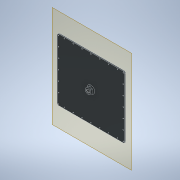
# Autodesk Inventor part: Крышка картера 2
Saved by Autodesk Inventor 2021 (Build 250183000, 183)
## iProperties
Created: 2020-12-12
Part Number: Крышка картера 2
Material: Чугун, серый
Document SubType Name: Modeling
Designer: Тимоха
Mass: 32984 g
Surface Area: 9566.62 cm^2
Volume: 4613.15 cm^3
Density: 7.15 g/cm^3
Appearance: Чугун серый
Author: Тимоха
Autodesk Inventor part; units mm, degrees
ref_plane "YZ Plane" through (0, 0, 0) normal (1, 0, 0) x (0, 1, 0)
ref_plane "XZ Plane" through (0, 0, 0) normal (0, 1, 0) x (-1, 0, 0)
ref_plane "XY Plane" through (0, 0, 0) normal (0, 0, 1) x (1, 0, 0)
ref_plane "РабПлоскость1" through (0, 0, 0) normal (0, 0, 1) x (1, 0, 0)
sketch "Эскиз1" plane through (0, 0, 0) normal (0, 0, 1) x (1, 0, 0)
  circle A0 centre (340, 472) radius 4 projected
  circle A1 centre (340, 367) radius 4 projected
  circle A2 centre (340, 322.8) radius 4 projected
  circle A3 centre (340, 218.5) radius 4 projected
  circle A4 centre (340, 114.2) radius 4 projected
  circle A5 centre (340, 9.9) radius 4 projected
  circle A6 centre (340, -94.4) radius 4 projected
  circle A7 centre (340, -198.7) radius 4 projected
  circle A8 centre (340, -303) radius 4 projected
  circle A9 centre (340, -347) radius 4 projected
  circle A10 centre (340, -407) radius 4 projected
  circle A11 centre (340, -467) radius 4 projected
  circle A12 centre (278, 472) radius 4 projected
  circle A13 centre (185, 472) radius 4 projected
  circle A14 centre (92, 472) radius 4 projected
  circle A15 centre (-1, 472) radius 4 projected
  circle A16 centre (-94, 472) radius 4 projected
  circle A17 centre (-187, 472) radius 4 projected
  circle A18 centre (-280, 472) radius 4 projected
  circle A19 centre (-340, 472) radius 4 projected
  circle A20 centre (-340, 367) radius 4 projected
  circle A21 centre (-340, 322.8) radius 4 projected
  circle A22 centre (-340, 218.5) radius 4 projected
  circle A23 centre (-340, 114.2) radius 4 projected
  circle A24 centre (-340, 9.9) radius 4 projected
  circle A25 centre (-340, -94.4) radius 4 projected
  circle A26 centre (-340, -198.7) radius 4 projected
  circle A27 centre (-340, -303) radius 4 projected
  circle A28 centre (-340, -347) radius 4 projected
  circle A29 centre (-340, -407) radius 4 projected
  circle A30 centre (-340, -467) radius 4 projected
  line L0 (165, -460) -> (165, -485) projected
  line L1 (185, -485) -> (165, -485) projected
  line L2 (185, -475) -> (185, -485) projected
  line L3 (185, -475) -> (380, -475) projected
  line L4 (380, 475) -> (350, 475) projected
  line L5 (350, 475) -> (350, 485) projected
  line L6 (-350, 485) -> (350, 485) projected
  line L7 (-350, 475) -> (-350, 485) projected
  line L8 (-350, 475) -> (-380, 475) projected
  line L9 (-380, -475) -> (-185, -475) projected
  line L10 (-185, -475) -> (-185, -485) projected
  line L11 (-165, -485) -> (-185, -485) projected
  line L12 (-165, -485) -> (-165, -460) projected
  line L13 (-165, -460) -> (-330, -460) projected
  line L14 (-330, 460) -> (-330, -460) projected
  line L15 (-330, 460) -> (330, 460) projected
  line L16 (330, -460) -> (330, 460) projected
  line L17 (330, -460) -> (165, -460) projected
  circle A31 centre (278, -303) radius 4 projected
  circle A32 centre (185, -303) radius 4 projected
  circle A33 centre (92, -303) radius 4 projected
  circle A34 centre (-1, -303) radius 4 projected
  circle A35 centre (-94, -303) radius 4 projected
  circle A36 centre (-187, -303) radius 4 projected
  circle A37 centre (-280, -303) radius 4 projected
  circle A38 centre (278, -347) radius 4 projected
  circle A39 centre (185, -347) radius 4 projected
  circle A40 centre (92, -347) radius 4 projected
  circle A41 centre (-1, -347) radius 4 projected
  circle A42 centre (-94, -347) radius 4 projected
  circle A43 centre (-187, -347) radius 4 projected
  circle A44 centre (-280, -347) radius 4 projected
  line L18 (-330, -291) -> (-330, -359) projected
  line L19 (-330, -359) -> (330, -359) projected
  line L20 (330, -291) -> (330, -359) projected
  line L21 (-330, -291) -> (330, -291) projected
  circle A45 centre (278, 367) radius 4 projected
  circle A46 centre (185, 367) radius 4 projected
  circle A47 centre (92, 367) radius 4 projected
  circle A48 centre (-1, 367) radius 4 projected
  circle A49 centre (-94, 367) radius 4 projected
  circle A50 centre (-187, 367) radius 4 projected
  circle A51 centre (-280, 367) radius 4 projected
  circle A52 centre (278, 323) radius 4 projected
  circle A53 centre (185, 323) radius 4 projected
  circle A54 centre (92, 323) radius 4 projected
  circle A55 centre (-1, 323) radius 4 projected
  circle A56 centre (-94, 323) radius 4 projected
  circle A57 centre (-187, 323) radius 4 projected
  circle A58 centre (-280, 323) radius 4 projected
  line L22 (-330, 379) -> (-330, 311) projected
  line L23 (-330, 311) -> (330, 311) projected
  line L24 (330, 379) -> (330, 311) projected
  line L25 (-330, 379) -> (330, 379) projected
  circle A59 centre (-340, 322.8) radius 14
  circle A60 centre (-340, -303) radius 14
  circle A61 centre (340, -303) radius 14
  circle A62 centre (340, 322.8) radius 14
  line L26 (340, 336.8) -> (-340, 336.8)
  line L27 (-354, 322.8) -> (-354, -303)
  line L28 (-340, -317) -> (340, -317)
  line L29 (354, -303) -> (354, 322.8)
  spline S0 degree 3 poles (-370, 316.7157) (-371.226, 316.7157) (-372.452, 316.5956) (-375.5798, 315.9798) (-377.4441, 315.3011) (-379.4493, 314.2131) (-379.7267, 314.0539) (-380, 313.8881) knots 25.431649 25.431649 25.431649 25.431649 25.799448 25.799448 26.387926 26.387926 26.483827 26.483827 26.483827 26.483827 projected
  spline S1 degree 3 poles (-360, 299.3952) (-360, 300.6696) (-360.1945, 302.0462) (-360.9458, 304.7063) (-361.4997, 305.9906) (-363.0323, 308.8381) (-364.2894, 310.5672) (-367.0866, 313.808) (-368.6145, 315.3302) (-370, 316.7157) knots 0 0 0 0 0.382316 0.382316 0.764632 0.764632 1.352446 1.352446 1.94026 1.94026 1.94026 1.94026 projected
  line L30 (-360, 299.3952) -> (-360, 277.9108) projected
  spline S2 degree 3 poles (-370, 260.5903) (-368.6145, 261.9758) (-367.0866, 263.498) (-364.2894, 266.7388) (-363.0323, 268.4679) (-361.4997, 271.3154) (-360.9458, 272.5997) (-360.1945, 275.2598) (-360, 276.6364) (-360, 277.9108) knots 5.055322 5.055322 5.055322 5.055322 5.643136 5.643136 6.230951 6.230951 6.613267 6.613267 6.995583 6.995583 6.995583 6.995583 projected
  spline S3 degree 3 poles (-380, 263.2891) (-378.6731, 262.5173) (-377.2567, 261.8994) (-373.9153, 260.8819) (-371.9577, 260.5903) (-370, 260.5903) knots 11.600008 11.600008 11.600008 11.600008 12.060517 12.060517 12.64782 12.64782 12.64782 12.64782 projected
  line L31 (-380, 263.2891) -> (-380, -243.2891) projected
  spline S4 degree 3 poles (-370, -240.5903) (-371.2894, -240.5903) (-372.5789, -240.7163) (-375.8683, -241.3651) (-377.8293, -242.082) (-379.7569, -243.1494) (-379.8788, -243.2186) (-380, -243.2891) knots 12.64782 12.64782 12.64782 12.64782 13.034648 13.034648 13.653574 13.653574 13.695631 13.695631 13.695631 13.695631 projected
  spline S5 degree 3 poles (-360, -257.9108) (-360, -256.6364) (-360.1945, -255.2598) (-360.9458, -252.5997) (-361.4997, -251.3154) (-363.0323, -248.4679) (-364.2894, -246.7388) (-367.0866, -243.498) (-368.6145, -241.9758) (-370, -240.5903) knots 0 0 0 0 0.382316 0.382316 0.764632 0.764632 1.352446 1.352446 1.94026 1.94026 1.94026 1.94026 projected
  line L32 (-360, -257.9108) -> (-360, -279.3952) projected
  spline S6 degree 3 poles (-370, -296.7157) (-368.6145, -295.3302) (-367.0866, -293.808) (-364.2894, -290.5672) (-363.0323, -288.8381) (-361.4997, -285.9906) (-360.9458, -284.7063) (-360.1945, -282.0462) (-360, -280.6696) (-360, -279.3952) knots 5.055322 5.055322 5.055322 5.055322 5.643136 5.643136 6.230951 6.230951 6.613267 6.613267 6.995583 6.995583 6.995583 6.995583 projected
  spline S7 degree 3 poles (-380, -293.8881) (-379.7267, -294.0539) (-379.4493, -294.2131) (-377.4441, -295.3011) (-375.5798, -295.9798) (-372.452, -296.5956) (-371.226, -296.7157) (-370, -296.7157) knots -1.052177 -1.052177 -1.052177 -1.052177 -0.956277 -0.956277 -0.367799 -0.367799 0 0 0 0 projected
  line L33 (-380, -293.8881) -> (-380, -356.1119) projected
  spline S8 degree 3 poles (-370, -353.2843) (-371.226, -353.2843) (-372.452, -353.4044) (-375.5798, -354.0202) (-377.4441, -354.6989) (-379.4493, -355.7869) (-379.7267, -355.9461) (-380, -356.1119) knots 12.715825 12.715825 12.715825 12.715825 13.083623 13.083623 13.672101 13.672101 13.768002 13.768002 13.768002 13.768002 projected
  spline S9 degree 3 poles (-360, -370.6048) (-360, -369.3304) (-360.1945, -367.9538) (-360.9458, -365.2937) (-361.4997, -364.0094) (-363.0323, -361.1619) (-364.2894, -359.4328) (-367.0866, -356.192) (-368.6145, -354.6698) (-370, -353.2843) knots 0 0 0 0 0.382316 0.382316 0.764632 0.764632 1.352446 1.352446 1.94026 1.94026 1.94026 1.94026 projected
  line L34 (-360, -370.6048) -> (-360, -392.0892) projected
  spline S10 degree 3 poles (-370, -409.4097) (-368.6145, -408.0242) (-367.0866, -406.502) (-364.2894, -403.2612) (-363.0323, -401.5321) (-361.4997, -398.6846) (-360.9458, -397.4003) (-360.1945, -394.7402) (-360, -393.3636) (-360, -392.0892) knots 5.055322 5.055322 5.055322 5.055322 5.643136 5.643136 6.230951 6.230951 6.613267 6.613267 6.995583 6.995583 6.995583 6.995583 projected
  spline S11 degree 3 poles (-380, -406.7109) (-379.8788, -406.7814) (-379.7569, -406.8506) (-377.8293, -407.918) (-375.8683, -408.6349) (-372.5789, -409.2837) (-371.2894, -409.4097) (-370, -409.4097) knots -1.047812 -1.047812 -1.047812 -1.047812 -1.005754 -1.005754 -0.386829 -0.386829 0 0 0 0 projected
  line L35 (-380, -406.7109) -> (-380, -475) projected
  line L36 (380, -475) -> (380, -406.7109) projected
  spline S12 degree 3 poles (370, -409.4097) (371.2894, -409.4097) (372.5789, -409.2837) (375.8683, -408.6349) (377.8293, -407.918) (379.7569, -406.8506) (379.8788, -406.7814) (380, -406.7109) knots 12.64782 12.64782 12.64782 12.64782 13.034648 13.034648 13.653574 13.653574 13.695631 13.695631 13.695631 13.695631 projected
  spline S13 degree 3 poles (360, -392.0892) (360, -393.3636) (360.1945, -394.7402) (360.9458, -397.4003) (361.4997, -398.6846) (363.0323, -401.5321) (364.2894, -403.2612) (367.0866, -406.502) (368.6145, -408.0242) (370, -409.4097) knots 0 0 0 0 0.382316 0.382316 0.764632 0.764632 1.352446 1.352446 1.94026 1.94026 1.94026 1.94026 projected
  line L37 (360, -392.0892) -> (360, -370.6048) projected
  spline S14 degree 3 poles (370, -353.2843) (368.6145, -354.6698) (367.0866, -356.192) (364.2894, -359.4328) (363.0323, -361.1619) (361.4997, -364.0094) (360.9458, -365.2937) (360.1945, -367.9538) (360, -369.3304) (360, -370.6048) knots 5.055322 5.055322 5.055322 5.055322 5.643136 5.643136 6.230951 6.230951 6.613267 6.613267 6.995583 6.995583 6.995583 6.995583 projected
  spline S15 degree 3 poles (380, -356.1119) (378.2451, -355.0477) (376.3252, -354.255) (372.9103, -353.4538) (371.4552, -353.2843) (370, -353.2843) knots -1.052177 -1.052177 -1.052177 -1.052177 -0.436564 -0.436564 0 0 0 0 projected
  line L38 (380, -356.1119) -> (380, -293.8881) projected
  spline S16 degree 3 poles (370, -296.7157) (371.226, -296.7157) (372.452, -296.5956) (375.5798, -295.9798) (377.4441, -295.3011) (379.4493, -294.2131) (379.7267, -294.0539) (380, -293.8881) knots 12.715825 12.715825 12.715825 12.715825 13.083623 13.083623 13.672101 13.672101 13.768002 13.768002 13.768002 13.768002 projected
  spline S17 degree 3 poles (360, -279.3952) (360, -280.6696) (360.1945, -282.0462) (360.9458, -284.7063) (361.4997, -285.9906) (363.0323, -288.8381) (364.2894, -290.5672) (367.0866, -293.808) (368.6145, -295.3302) (370, -296.7157) knots 0 0 0 0 0.382316 0.382316 0.764632 0.764632 1.352446 1.352446 1.94026 1.94026 1.94026 1.94026 projected
  line L39 (360, -279.3952) -> (360, -257.9108) projected
  spline S18 degree 3 poles (370, -240.5903) (368.6145, -241.9758) (367.0866, -243.498) (364.2894, -246.7388) (363.0323, -248.4679) (361.4997, -251.3154) (360.9458, -252.5997) (360.1945, -255.2598) (360, -256.6364) (360, -257.9108) knots 5.055322 5.055322 5.055322 5.055322 5.643136 5.643136 6.230951 6.230951 6.613267 6.613267 6.995583 6.995583 6.995583 6.995583 projected
  spline S19 degree 3 poles (380, -243.2891) (378.6731, -242.5173) (377.2567, -241.8994) (373.9153, -240.8819) (371.9577, -240.5903) (370, -240.5903) knots 11.600008 11.600008 11.600008 11.600008 12.060517 12.060517 12.64782 12.64782 12.64782 12.64782 projected
  line L40 (380, -243.2891) -> (380, 263.2891) projected
  spline S20 degree 3 poles (370, 260.5903) (371.2894, 260.5903) (372.5789, 260.7163) (375.8683, 261.3651) (377.8293, 262.082) (379.7569, 263.1494) (379.8788, 263.2186) (380, 263.2891) knots 25.295639 25.295639 25.295639 25.295639 25.682468 25.682468 26.301393 26.301393 26.343451 26.343451 26.343451 26.343451 projected
  spline S21 degree 3 poles (360, 277.9108) (360, 276.6364) (360.1945, 275.2598) (360.9458, 272.5997) (361.4997, 271.3154) (363.0323, 268.4679) (364.2894, 266.7388) (367.0866, 263.498) (368.6145, 261.9758) (370, 260.5903) knots 0 0 0 0 0.382316 0.382316 0.764632 0.764632 1.352446 1.352446 1.94026 1.94026 1.94026 1.94026 projected
  line L41 (360, 277.9108) -> (360, 299.3952) projected
  spline S22 degree 3 poles (370, 316.7157) (368.6145, 315.3302) (367.0866, 313.808) (364.2894, 310.5672) (363.0323, 308.8381) (361.4997, 305.9906) (360.9458, 304.7063) (360.1945, 302.0462) (360, 300.6696) (360, 299.3952) knots 5.055322 5.055322 5.055322 5.055322 5.643136 5.643136 6.230951 6.230951 6.613267 6.613267 6.995583 6.995583 6.995583 6.995583 projected
  spline S23 degree 3 poles (380, 313.8881) (379.7267, 314.0539) (379.4493, 314.2131) (377.4441, 315.3011) (375.5798, 315.9798) (372.452, 316.5956) (371.226, 316.7157) (370, 316.7157) knots -1.052177 -1.052177 -1.052177 -1.052177 -0.956277 -0.956277 -0.367799 -0.367799 0 0 0 0 projected
  line L42 (380, 313.8881) -> (380, 376.1119) projected
  spline S24 degree 3 poles (370, 373.2843) (371.226, 373.2843) (372.452, 373.4044) (375.5798, 374.0202) (377.4441, 374.6989) (379.4493, 375.7869) (379.7267, 375.9461) (380, 376.1119) knots 25.431649 25.431649 25.431649 25.431649 25.799448 25.799448 26.387926 26.387926 26.483827 26.483827 26.483827 26.483827 projected
  spline S25 degree 3 poles (360, 390.6048) (360, 389.3304) (360.1945, 387.9538) (360.9458, 385.2937) (361.4997, 384.0094) (363.0323, 381.1619) (364.2894, 379.4328) (367.0866, 376.192) (368.6145, 374.6698) (370, 373.2843) knots 0 0 0 0 0.382316 0.382316 0.764632 0.764632 1.352446 1.352446 1.94026 1.94026 1.94026 1.94026 projected
  line L43 (360, 390.6048) -> (360, 412.0892) projected
  spline S26 degree 3 poles (370, 429.4097) (368.6145, 428.0242) (367.0866, 426.502) (364.2894, 423.2612) (363.0323, 421.5321) (361.4997, 418.6846) (360.9458, 417.4003) (360.1945, 414.7402) (360, 413.3636) (360, 412.0892) knots 5.055322 5.055322 5.055322 5.055322 5.643136 5.643136 6.230951 6.230951 6.613267 6.613267 6.995583 6.995583 6.995583 6.995583 projected
  spline S27 degree 3 poles (380, 426.7109) (378.6731, 427.4827) (377.2567, 428.1006) (373.9153, 429.1181) (371.9577, 429.4097) (370, 429.4097) knots -1.047812 -1.047812 -1.047812 -1.047812 -0.587302 -0.587302 0 0 0 0 projected
  line L44 (380, 426.7109) -> (380, 475) projected
  line L45 (-380, 475) -> (-380, 426.7109) projected
  spline S28 degree 3 poles (-370, 429.4097) (-371.2894, 429.4097) (-372.5789, 429.2837) (-375.8683, 428.6349) (-377.8293, 427.918) (-379.7569, 426.8506) (-379.8788, 426.7814) (-380, 426.7109) knots 12.64782 12.64782 12.64782 12.64782 13.034648 13.034648 13.653574 13.653574 13.695631 13.695631 13.695631 13.695631 projected
  spline S29 degree 3 poles (-360, 412.0892) (-360, 413.3636) (-360.1945, 414.7402) (-360.9458, 417.4003) (-361.4997, 418.6846) (-363.0323, 421.5321) (-364.2894, 423.2612) (-367.0866, 426.502) (-368.6145, 428.0242) (-370, 429.4097) knots 0 0 0 0 0.382316 0.382316 0.764632 0.764632 1.352446 1.352446 1.94026 1.94026 1.94026 1.94026 projected
  line L46 (-360, 412.0892) -> (-360, 390.6048) projected
  spline S30 degree 3 poles (-370, 373.2843) (-368.6145, 374.6698) (-367.0866, 376.192) (-364.2894, 379.4328) (-363.0323, 381.1619) (-361.4997, 384.0094) (-360.9458, 385.2937) (-360.1945, 387.9538) (-360, 389.3304) (-360, 390.6048) knots 5.055322 5.055322 5.055322 5.055322 5.643136 5.643136 6.230951 6.230951 6.613267 6.613267 6.995583 6.995583 6.995583 6.995583 projected
  spline S31 degree 3 poles (-380, 376.1119) (-379.7267, 375.9461) (-379.4493, 375.7869) (-377.4441, 374.6989) (-375.5798, 374.0202) (-372.452, 373.4044) (-371.226, 373.2843) (-370, 373.2843) knots -1.052177 -1.052177 -1.052177 -1.052177 -0.956277 -0.956277 -0.367799 -0.367799 0 0 0 0 projected
  line L47 (-380, 376.1119) -> (-380, 313.8881) projected
  point P0 (0, 0)
  dimension "d0" = 10
  dimension "d1" = 10
  dimension "d2" = 10
  dimension "d3" = 10
  constraints: 8 end point, 8 point on circle, 5 tangent, 4 centre point
  measures "d0" radial gap between concentric circles of A21 A59
  measures "d1" radial gap between concentric circles of A27 A60
  measures "d2" radial gap between concentric circles of A8 A61
  measures "d3" radial gap between concentric circles of A2 A62
extrude "Выдавливание1" add sketch "Эскиз1" along normal blind 10 contours L28 L14 A60 L21 L16 A61 | L16 A61 L28 | A61 L16 | L16 A61 | L28 A60 L14 | L16 A62 L29 A61 | A60 L14 | L14 A60 | L21 L14 L23 L16 | A60 L27 A59 L14 | A62 L16 | L23 L14 A59 L26 L16 A62 | A59 L14 | A62 L16 L26 | A62 L16 | L26 L14 A59 | L14 A59
sketch "Эскиз2" plane through (0, 0, 10) normal (0, 0, 1) x (1, 0, 0)
  circle A0 centre (0, 0) radius 30
  dimension "d6" = 60
  constraints: 1 centre point, 1 coincident
  measures "d6" diameter of A0
extrude "Выдавливание2" add sketch "Эскиз2" along normal blind 30
fillet "Сопряжение1" radius 10 1 edges at (-30, 0, 10)
sketch "Эскиз3" plane through (0, 0, 40) normal (0, 0, 1) x (1, 0, 0)
  circle A0 centre (0, 0) radius 15
  dimension "d10" = 30
  constraints: 1 centre point, 1 coincident
  measures "d10" diameter of A0
extrude "Выдавливание3" cut sketch "Эскиз3" against normal through all
thread "Резьба1" size "M30x3.5" class "6H" standard "ANSI Metric M Profile" full length
chamfer "Фаска1" distance 2 angle 45 2 edges at (-15, 0, 40) (-15, 0, 0)
